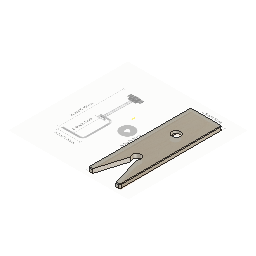
Jewelry Sawing Block (Autodesk Fusion 360 design; units mm, degrees)
Autodesk Fusion 360 part; units mm, degrees
sketch "Sketch1" plane through (0, 0, 0) normal (0, 0, 1) x (1, 0, 0) in component "Jewelry Sawing Block"
  line L0 (-30, 97.5) -> (30, 97.5)
  line L1 (30, 97.5) -> (30, -97.5)
  line L2 (30, -97.5) -> (-30, -97.5)
  line L3 (-30, -97.5) -> (-30, 97.5)
  line L4 (-30, 97.5) -> (30, -97.5) construction
  line L5 (30, 97.5) -> (-30, -97.5) construction
  circle A0 centre (0, 40) radius 8
  line L6 (0, 0) -> (0, 40) construction
  line L7 (-8, 97.5) -> (-8, 40)
  line L8 (8, 97.5) -> (8, 40)
  circle A1 centre (0, -35) radius 8
  line L9 (0, 0) -> (0, -35) construction
  line L10 (-22.5, -97.5) -> (-5.5, -40.8095)
  line L11 (22.5, -97.5) -> (5.5, -40.8095)
  dimension "d1" = 195
  dimension "d2" = 60
  dimension "d3" = 16
  dimension "d4" = 40
  dimension "d5" = 16
  dimension "d6" = 35
  dimension "d7" = 7.5
  dimension "d8" = 11
  constraint horizontal L0
  constraint perpendicular L0 L1
  constraint parallel L0 L2
  constraint parallel L1 L3
  constraint coincident L4 L6.start
  constraint coincident L5 L6.start
  constraint coincident L6.start L9.start
  constraint vertical L6
  constraint coincident A0.centre L6.end
  constraint coincident L0 L7.start
  constraint coincident A0 L7.end
  constraint perpendicular L0 L7
  constraint symmetric L6 L7.start L8.start
  constraint symmetric L6 L7.end L8.end
  constraint tangent A0 L7
  constraint coincident A1.centre L9.end
  constraint vertical L9
  constraint coincident L2 L10.start
  constraint coincident A1 L10.end
  constraint symmetric L9 L10.start L11.start
  constraint symmetric L9 L10.end L11.end
  measures "d1" distance of L0.start L2.end
  measures "d2" distance of L0.start L0.end
  measures "d3" diameter of A0
  measures "d4" distance of L6.start A0.centre
  measures "d5" diameter of A1
  measures "d6" vertical distance of A1.centre L6.start
  measures "d7" distance of L2.end L10.start
  measures "d8" distance of L10.end L11.end
extrude "Extrude1" add sketch "Sketch1" along normal blind 8 contours L0 L1 L2 L3 A0 L7 L8 A1 L10 L11 | L0 A0 L7 L8 in component "Jewelry Sawing Block"
extrude "Extrude2" cut sketch "Sketch1" along normal blind 3 contours L0 A0 L7 L8 in component "Jewelry Sawing Block"
fillet "Fillet1" radius 3 4 edges at (-30, -97.5, 4) (30, -97.5, 4) (30, 97.5, 4) (-30, 97.5, 4) in component "Jewelry Sawing Block"
chamfer "Chamfer1" distance 1 angle 45 19 edges at (30, 0, 0) (29.1213, -96.6213, 0) (24.75, -97.5, 0) (17.5, 97.5, 0) (29.1213, 96.6213, 0) (-30, 0, 0) (-29.1213, 96.6213, 0) (-17.5, 97.5, 0) (-24.75, -97.5, 0) (-29.1213, -96.6213, 0) (30, 0, 8) (29.1213, 96.6213, 8) (0, 97.5, 8) (-29.1213, 96.6213, 8) (-30, 0, 8) (-29.1213, -96.6213, 8) (-24.75, -97.5, 8) (24.75, -97.5, 8) (29.1213, -96.6213, 8) in component "Jewelry Sawing Block"
component "Jewelry Sawing Block" placed x (1, 0, 0) y (0, 1, 0) z (0, 0, 1) at (0, 0, 0)
named bodies: "Jewelry Sawing Block"
